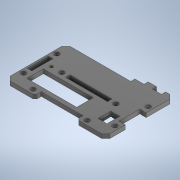
# Autodesk Inventor part: Cockpit_side_frame
Saved by Autodesk Inventor 2020.4 (Build 244396000, 396)
## iProperties
Created: 2022-01-04
Part Number: Cockpit_side_frame
Material: アセタール樹脂、黒
Document SubType Name: Modeling
Designer: Masato Kubotera
Density: 1.425 g/cm^3
Appearance: 滑らか - 黒
Mass: 55.613 g
Surface Area: 192.228 cm^2
Volume: 39.0267 cm^3
Author: Masato Kubotera
Autodesk Inventor part; units mm, degrees
ref_plane "YZ Plane" through (0, 0, 0) normal (1, 0, 0) x (0, 1, 0)
ref_plane "XZ Plane" through (0, 0, 0) normal (0, 1, 0) x (-1, 0, 0)
ref_plane "XY Plane" through (0, 0, 0) normal (0, 0, 1) x (1, 0, 0)
sketch "スケッチ1" plane through (0, 0, 0) normal (0, 1, 0) x (-1, 0, 0)
  line L0 (-60, 36) -> (60, 36) construction
  line L1 (60, 36) -> (60, -36) construction
  line L2 (60, -36) -> (-60, -36) construction
  line L3 (-60, -36) -> (-60, 36) construction
  line L4 (-60, 36) -> (60, -36) construction
  line L5 (60, 36) -> (-60, -36) construction
  line L6 (-52.5, 6) -> (52.5, 6) construction
  line L7 (52.5, 6) -> (52.5, 1) construction
  line L8 (52.5, 1) -> (-52.5, 1) construction
  line L9 (-52.5, 1) -> (-52.5, 6) construction
  line L10 (-52.5, 6) -> (52.5, 1) construction
  line L11 (52.5, 6) -> (-52.5, 1) construction
  line L12 (0, 36) -> (0, -36) construction
  line L13 (-57.5, 33.5) -> (-52.5, 33.5) construction
  line L14 (-52.5, 33.5) -> (-52.5, -33.5) construction
  line L15 (-52.5, -33.5) -> (-57.5, -33.5) construction
  line L16 (-57.5, -33.5) -> (-57.5, 33.5) construction
  line L17 (-57.5, 33.5) -> (-52.5, -33.5) construction
  line L18 (-52.5, 33.5) -> (-57.5, -33.5) construction
  line L19 (-55, 36) -> (-60, 31)
  line L20 (-60, 0) -> (60, 0) construction
  line L21 (-46.5, 41) -> (32.5, 41) construction
  line L22 (32.5, 41) -> (32.5, 11) construction
  line L23 (32.5, 11) -> (-46.5, 11) construction
  line L24 (-46.5, 11) -> (-46.5, 41) construction
  line L25 (-46.5, 41) -> (32.5, 11) construction
  line L26 (32.5, 41) -> (-46.5, 11) construction
  line L27 (-55, -36) -> (-60, -31)
  line L28 (-60, 31) -> (-60, -31)
  line L29 (55, -36) -> (60, -31)
  line L30 (-52.5, -28.5) -> (52.5, -28.5) construction
  line L31 (52.5, -28.5) -> (52.5, -33.5) construction
  line L32 (52.5, -33.5) -> (-52.5, -33.5) construction
  line L33 (-52.5, -33.5) -> (-52.5, -28.5) construction
  line L34 (-52.5, -28.5) -> (52.5, -33.5) construction
  line L35 (52.5, -28.5) -> (-52.5, -33.5) construction
  line L36 (-25, -28.5) -> (-25, -33.5) construction
  line L37 (-55, -33.5) -> (-55, 33.5) construction
  line L38 (-57.5, 12.5) -> (-52.5, 12.5) construction
  line L39 (-57.55, 12.55) -> (-52.45, 12.55)
  line L40 (-52.45, 12.55) -> (-52.45, -12.55)
  line L41 (-52.45, -12.55) -> (-57.55, -12.55)
  line L42 (-57.55, -12.55) -> (-57.55, 12.55)
  line L43 (-57.55, 12.55) -> (-52.45, -12.55) construction
  line L44 (-52.45, 12.55) -> (-57.55, -12.55) construction
  arc A0 (-52.45, 11.0651) -> (-53.9349, 12.55) centre (-53.1925, 11.8075) ccw
  circle A1 centre (-55, 20) radius 1.6
  circle A2 centre (-55, -20) radius 1.6
  arc A3 (-53.9349, -12.55) -> (-52.45, -11.0651) centre (-53.1925, -11.8075) ccw
  line L45 (-57.5, -12.5) -> (-52.5, -12.5) construction
  arc A4 (-56.0651, 12.55) -> (-57.55, 11.0651) centre (-56.8075, 11.8075) ccw
  arc A5 (-57.55, -11.0651) -> (-56.0651, -12.55) centre (-56.8075, -11.8075) ccw
  line L46 (-52.5, -31) -> (52.5, -31) construction
  line L47 (-25.05, -33.5) -> (-25.05, -28.45)
  line L48 (-25.05, -28.45) -> (25.05, -28.45)
  circle A6 centre (-32.5, -31) radius 1.6
  circle A7 centre (32.5, -31) radius 1.6
  line L49 (25, -28.5) -> (25, -33.5) construction
  line L50 (52.5, 33.5) -> (57.5, 33.5) construction
  line L51 (57.5, 33.5) -> (57.5, -33.5) construction
  line L52 (57.5, -33.5) -> (52.5, -33.5) construction
  line L53 (52.5, -33.5) -> (52.5, 33.5) construction
  line L54 (52.5, 33.5) -> (57.5, -33.5) construction
  line L55 (57.5, 33.5) -> (52.5, -33.5) construction
  line L56 (52.5, 0) -> (57.5, 0) construction
  line L57 (52.5, -12.5) -> (57.5, -12.5) construction
  line L58 (55, -33.5) -> (55, 33.5) construction
  circle A8 centre (55, -20) radius 1.6
  line L59 (60, -12.55) -> (52.45, -12.55)
  line L60 (52.45, -12.55) -> (52.45, 12.55)
  arc A9 (52.45, -11.0651) -> (53.9349, -12.55) centre (53.1925, -11.8075) ccw
  line L61 (52.5, 12.5) -> (57.5, 12.5) construction
  circle A10 centre (55, 20) radius 1.6
  line L62 (60, 12.55) -> (52.45, 12.55)
  arc A11 (53.9349, 12.55) -> (52.45, 11.0651) centre (53.1925, 11.8075) ccw
  arc A12 (-23.5651, -28.45) -> (-25.05, -29.9349) centre (-24.3075, -29.1925) ccw
  arc A13 (25.05, -29.9349) -> (23.5651, -28.45) centre (24.3075, -29.1925) ccw
  circle A14 centre (-55, 20) radius 3
  circle A15 centre (-32.5, -31) radius 3
  circle A16 centre (-55, -20) radius 3
  circle A17 centre (32.5, -31) radius 3
  line L63 (-25.05, -33.5) -> (-27.55, -36)
  line L64 (-55, -36) -> (-27.55, -36)
  line L65 (25.05, -33.5) -> (25.05, -28.45)
  line L66 (25.05, -33.5) -> (27.55, -36)
  line L67 (55, -36) -> (27.55, -36)
  line L68 (25.05, 6.05) -> (-25.05, 6.05)
  line L69 (-25.05, 6.05) -> (-25.05, 0.95)
  line L70 (-25.05, 0.95) -> (25.05, 0.95)
  line L71 (25.05, 0.95) -> (25.05, 6.05)
  line L72 (25.05, 6.05) -> (-25.05, 0.95) construction
  line L73 (-25.05, 6.05) -> (25.05, 0.95) construction
  line L74 (-25, 6) -> (-25, 1) construction
  arc A18 (-23.5651, 6.05) -> (-25.05, 4.5651) centre (-24.3075, 5.3075) ccw
  line L75 (52.5, 3.5) -> (-52.5, 3.5) construction
  circle A19 centre (-32.5, 3.5) radius 1.6
  line L76 (25, 6) -> (25, 1) construction
  arc A20 (25.05, 4.5651) -> (23.5651, 6.05) centre (24.3075, 5.3075) ccw
  circle A21 centre (32.5, 3.5) radius 1.6
  arc A22 (-25.05, 2.4349) -> (-23.5651, 0.95) centre (-24.3075, 1.6925) ccw
  arc A23 (23.5651, 0.95) -> (25.05, 2.4349) centre (24.3075, 1.6925) ccw
  line L77 (60, 31) -> (60, 12.55)
  line L78 (60, -12.55) -> (60, -31)
  circle A24 centre (-32.5, 3.5) radius 3
  circle A25 centre (55, -20) radius 3
  circle A26 centre (55, 20) radius 3
  circle A27 centre (32.5, 3.5) radius 3
  line L79 (60, 31) -> (60, 41)
  line L80 (18, 36) -> (-55, 36)
  line L81 (60, 41) -> (55, 46)
  line L82 (55, 46) -> (50, 46)
  line L83 (50, 46) -> (50, 41)
  line L84 (50, 41) -> (39, 41)
  line L85 (39, 41) -> (39, 46)
  line L86 (39, 46) -> (29, 46)
  line L87 (29, 46) -> (29, 41)
  line L88 (29, 41) -> (18, 41)
  line L89 (18, 41) -> (18, 36)
  circle A28 centre (-45, 3.5) radius 1.75
  line L90 (34, 46) -> (34, 41) construction
  line L91 (37.9, -7.85) -> (47.1, -7.85) construction
  line L92 (47.1, -7.85) -> (47.1, -21.65) construction
  line L93 (47.1, -21.65) -> (37.9, -21.65) construction
  line L94 (37.9, -21.65) -> (37.9, -7.85) construction
  line L95 (37.9, -7.85) -> (47.1, -21.65) construction
  line L96 (47.1, -7.85) -> (37.9, -21.65) construction
  line L97 (37.2, -7.2) -> (47.8, -7.2) construction
  line L98 (47.8, -7.2) -> (47.8, -22.3) construction
  line L99 (47.8, -22.3) -> (37.2, -22.3) construction
  line L100 (37.2, -22.3) -> (37.2, -7.2) construction
  line L101 (37.2, -7.2) -> (47.8, -22.3) construction
  line L102 (47.8, -7.2) -> (37.2, -22.3) construction
  line L103 (42.5, -7.2) -> (42.5, -22.3) construction
  line L104 (47.8, -14.75) -> (37.2, -14.75) construction
  line L105 (38.6349, -7.15) -> (46.3651, -7.15)
  line L106 (37.15, -8.6349) -> (37.15, -20.8651)
  line L107 (39.3349, -7.8) -> (45.6651, -7.8)
  line L108 (37.85, -9.2849) -> (37.85, -20.2151)
  arc A29 (38.6349, -7.15) -> (37.15, -8.6349) centre (37.8925, -7.8925) ccw
  arc A30 (39.3349, -7.8) -> (37.85, -9.2849) centre (38.5925, -8.5425) ccw
  arc A31 (47.85, -8.6349) -> (46.3651, -7.15) centre (47.1075, -7.8925) ccw
  arc A32 (47.15, -9.2849) -> (45.6651, -7.8) centre (46.4075, -8.5425) ccw
  line L109 (38.6349, -22.35) -> (46.3651, -22.35)
  line L110 (39.3349, -21.7) -> (45.6651, -21.7)
  arc A33 (37.15, -20.8651) -> (38.6349, -22.35) centre (37.8925, -21.6075) ccw
  arc A34 (37.85, -20.2151) -> (39.3349, -21.7) centre (38.5925, -20.9575) ccw
  arc A35 (46.3651, -22.35) -> (47.85, -20.8651) centre (47.1075, -21.6075) ccw
  arc A36 (45.6651, -21.7) -> (47.15, -20.2151) centre (46.4075, -20.9575) ccw
  line L111 (47.85, -8.6349) -> (47.85, -20.8651)
  line L112 (47.15, -9.2849) -> (47.15, -20.2151)
  line L113 (-47.5, -3.5) -> (12.5, -3.5)
  line L114 (12.5, -3.5) -> (12.5, -23.5)
  line L115 (12.5, -23.5) -> (-47.5, -23.5)
  line L116 (-47.5, -23.5) -> (-47.5, -3.5)
  line L117 (-47.5, -3.5) -> (12.5, -23.5) construction
  line L118 (12.5, -3.5) -> (-47.5, -23.5) construction
  point P0 (0, 0)
  point P1 (0, 3.5)
  point P2 (-55, 0)
  point P3 (-55, 0)
  point P4 (-7, 26)
  point P5 (0, -31)
  point P6 (0, 3.5)
  point P7 (25.05, 2.4349)
  point P8 (23.5651, 0.95)
  point P9 (-23.5651, 0.95)
  point P10 (-25.05, 2.4349)
  point P11 (23.5651, 6.05)
  point P12 (25.05, 4.5651)
  point P13 (-57.55, -11.0651)
  point P14 (-57.55, 11.0651)
  point P15 (-56.0651, 12.55)
  point P16 (-52.45, -11.0651)
  point P17 (-53.9349, -12.55)
  point P18 (-56.0651, -12.55)
  point P19 (42.5, -14.75)
  point P20 (37.15, -7.15)
  point P21 (37.85, -7.8)
  point P22 (-17.5, -13.5)
  dimension "d0" = 72
  dimension "d1" = 120
  dimension "d3" = 5
  dimension "d4" = 5
  dimension "d6" = 5
  dimension "d7" = 5
  dimension "d8" = 79
  dimension "d9" = 6
  dimension "d11" = 5
  dimension "d12" = 1.05
  dimension "d13" = 3.2
  dimension "d14" = 40
  dimension "d15" = 25
  dimension "d16" = 0.05
  dimension "d17" = 0.05
  dimension "d18" = 3.2
  dimension "d19" = 50
  dimension "d20" = 0.05
  dimension "d21" = 0.05
  dimension "d23" = 65
  dimension "d24" = 5
  dimension "d25" = 30
  dimension "d28" = 3.2
  dimension "d29" = 1.05
  dimension "d30" = 0.05
  dimension "d31" = 0.05
  dimension "d32" = 40
  dimension "d33" = 25
  dimension "d34" = 105
  dimension "d35" = 1.05
  dimension "d36" = 5
  dimension "d37" = 5
  dimension "d38" = 6
  dimension "d39" = 6
  dimension "d40" = 2.5
  dimension "d41" = 1.05
  dimension "d42" = 3.2
  dimension "d43" = 50
  dimension "d44" = 0.05
  dimension "d45" = 0.05
  dimension "d46" = 65
  dimension "d47" = 29.5
  dimension "d48" = 2.5
  dimension "d51" = 6
  dimension "d52" = 6
  dimension "d55" = 67
  dimension "d63" = 20
  dimension "d64" = 5
  dimension "d65" = 10
  dimension "d66" = 3.5
  dimension "d69" = 32.5
  dimension "d70" = 10
  dimension "d72" = 5
  dimension "d73" = 5
  dimension "d74" = 10
  dimension "d75" = 16
  dimension "d76" = 78
  dimension "d77" = 9.2
  dimension "d78" = 13.8
  dimension "d79" = 10.6
  dimension "d80" = 15.1
  dimension "d84" = 1.05
  dimension "d85" = 0.05
  dimension "d86" = 0.05
  constraints: 238 end point, 68 symmetric about line, 47 point on circle, 42 midpoint, 40 point on line, 37 centre point, 29 parallel, 22 perpendicular, 11 horizontal, 9 collinear, 4 coincident, 3 vertical, 22 other
  measures "d0" distance of L0.end L1.end
  measures "d1" distance of L0.start L0.end
  measures "d3" distance of L6.end L7.end
  measures "d4" distance of L13.start L13.end
  measures "d6" distance of L0.start L19.start
  measures "d7" distance of L19.end L0.start
  measures "d8" distance of L21.start L21.end
  measures "d9" distance between parallel lines of L14 L24
  measures "d11" distance of L30.end L31.end
  measures "d12" radius of A0
  measures "d13" diameter of A1
  measures "d14" distance of A2.centre A1.centre
  measures "d15" distance between parallel lines of L45 L38
  measures "d16" distance between parallel lines of L38 L39
  measures "d17" distance between parallel lines of L42 L16
  measures "d18" diameter of A6
  measures "d19" distance of L49.end L36.end
  measures "d20" distance between parallel lines of L47 L36
  measures "d21" distance between parallel lines of L30 L48
  measures "d23" distance of A7.centre A6.centre
  measures "d24" distance of L51.end L52.end
  measures "d25" distance of L21.end L22.end
  measures "d28" diameter of A8
  measures "d29" radius of A9
  measures "d30" distance between parallel lines of L60 L53
  measures "d31" distance between parallel lines of L61 L62
  measures "d32" distance of A8.centre A10.centre
  measures "d33" distance between parallel lines of L57 L61
  measures "d34" distance of L7.end L8.end
  measures "d35" radius of A12
  measures "d36" distance between parallel lines of L21 L0
  measures "d37" distance between parallel lines of L6 L23
  measures "d38" diameter of A14
  measures "d39" diameter of A15
  measures "d40" horizontal distance of L47.start L63.end
  measures "d41" radius of A18
  measures "d42" diameter of A19
  measures "d43" distance between parallel lines of L76 L74
  measures "d44" distance between parallel lines of L69 L74
  measures "d45" distance between parallel lines of L68 L6
  measures "d46" distance of A21.centre A19.centre
  measures "d47" distance of L30.start L8.end
  measures "d48" horizontal distance of L50.end L0.end
  measures "d51" diameter of A24
  measures "d52" diameter of A25
  measures "d55" distance of L15.end L13.start
  measures "d63" distance between parallel lines of L22 L53
  measures "d64" distance of L86.end L87.end
  measures "d65" vertical distance of L80.start L86.end
  measures "d66" diameter of A28
  measures "d69" vertical distance of A28.centre L0.start
  measures "d70" distance of L85.end L86.end
  measures "d72" horizontal distance of L79.end L81.end
  measures "d73" horizontal distance of L79.end L81.end
  measures "d74" horizontal distance of L82.end L79.end
  measures "d75" horizontal distance of L88.end L90.start
  measures "d76" horizontal distance of L0.start L88.end
  measures "d77" distance of L92.end L93.end
  measures "d78" distance of L91.end L92.end
  measures "d79" distance of L98.end L99.end
  measures "d80" distance of L97.end L98.end
  measures "d84" radius of A29
  measures "d85" distance between parallel lines of L97 L105
  measures "d86" distance between parallel lines of L106 L100
extrude "押し出し1" add sketch "スケッチ1" along normal blind 5 contours L80 L89 L88 L87 L86 L85 L84 L83 L82 L81 L79 L77 L62 A11 L60 A9 L59 L78 L29 L67 L66 L65 A13 L48 A12 L47 L63 L64 L27 L28 L19
extrude "押し出し2" add sketch "スケッチ1" along normal blind 3.5 contours A14 | A15 | A16 | A17 | A24 | A25 | A26 | A27
extrude "押し出し3" add sketch "スケッチ1" along normal blind 2 contours L105 A31 L111 A35 L109 A33 L106 A29
equation "\"d7\" = d6"
equation "\"d18\" = d13"
equation "\"d20\" = d16"
equation "\"d21\" = d20"
equation "\"d29\" = d12"
equation "\"d30\" = d16"
equation "\"d31\" = d30"
equation "\"d35\" = d12"
